Autodesk Inventor part; units mm, degrees
(part 3 of 3)
  circle A2075 centre (2.45, 2.35) radius 0.15
  circle A2076 centre (2.45, 2.05) radius 0.15
  circle A2077 centre (2.45, 1.75) radius 0.15
  circle A2078 centre (2.45, 1.45) radius 0.15
  circle A2079 centre (2.45, 1.15) radius 0.15
  circle A2080 centre (2.45, 0.85) radius 0.15
  circle A2081 centre (2.45, 0.55) radius 0.15
  circle A2082 centre (2.45, 0.25) radius 0.15
  circle A2083 centre (2.45, -0.05) radius 0.15
  circle A2084 centre (2.45, -0.35) radius 0.15
  circle A2085 centre (2.45, -0.65) radius 0.15
  circle A2086 centre (2.45, -0.95) radius 0.15
  circle A2087 centre (2.45, -1.25) radius 0.15
  circle A2088 centre (2.45, -1.55) radius 0.15
  circle A2089 centre (2.45, -1.85) radius 0.15
  circle A2090 centre (2.45, -2.15) radius 0.15
  circle A2091 centre (2.45, -2.45) radius 0.15
  circle A2092 centre (2.45, -2.75) radius 0.15
  circle A2093 centre (2.45, -3.05) radius 0.15
  circle A2094 centre (2.45, -3.35) radius 0.15
  circle A2095 centre (2.45, -3.65) radius 0.15
  circle A2096 centre (2.45, -3.95) radius 0.15
  circle A2097 centre (2.45, -4.25) radius 0.15
  circle A2098 centre (2.45, -4.55) radius 0.15
  circle A2099 centre (2.45, -4.85) radius 0.15
  circle A2100 centre (2.75, 9.85) radius 0.15
  circle A2101 centre (2.75, 9.55) radius 0.15
  circle A2102 centre (2.75, 9.25) radius 0.15
  circle A2103 centre (2.75, 8.95) radius 0.15
  circle A2104 centre (2.75, 8.65) radius 0.15
  circle A2105 centre (2.75, 8.35) radius 0.15
  circle A2106 centre (2.75, 8.05) radius 0.15
  circle A2107 centre (2.75, 7.75) radius 0.15
  circle A2108 centre (2.75, 7.45) radius 0.15
  circle A2109 centre (2.75, 7.15) radius 0.15
  circle A2110 centre (2.75, 6.85) radius 0.15
  circle A2111 centre (2.75, 6.55) radius 0.15
  circle A2112 centre (2.75, 6.25) radius 0.15
  circle A2113 centre (2.75, 5.95) radius 0.15
  circle A2114 centre (2.75, 5.65) radius 0.15
  circle A2115 centre (2.75, 5.35) radius 0.15
  circle A2116 centre (2.75, 5.05) radius 0.15
  circle A2117 centre (2.75, 4.75) radius 0.15
  circle A2118 centre (2.75, 4.45) radius 0.15
  circle A2119 centre (2.75, 4.15) radius 0.15
  circle A2120 centre (2.75, 3.85) radius 0.15
  circle A2121 centre (2.75, 3.55) radius 0.15
  circle A2122 centre (2.75, 3.25) radius 0.15
  circle A2123 centre (2.75, 2.95) radius 0.15
  circle A2124 centre (2.75, 2.65) radius 0.15
  circle A2125 centre (2.75, 2.35) radius 0.15
  circle A2126 centre (2.75, 2.05) radius 0.15
  circle A2127 centre (2.75, 1.75) radius 0.15
  circle A2128 centre (2.75, 1.45) radius 0.15
  circle A2129 centre (2.75, 1.15) radius 0.15
  circle A2130 centre (2.75, 0.85) radius 0.15
  circle A2131 centre (2.75, 0.55) radius 0.15
  circle A2132 centre (2.75, 0.25) radius 0.15
  circle A2133 centre (2.75, -0.05) radius 0.15
  circle A2134 centre (2.75, -0.35) radius 0.15
  circle A2135 centre (2.75, -0.65) radius 0.15
  circle A2136 centre (2.75, -0.95) radius 0.15
  circle A2137 centre (2.75, -1.25) radius 0.15
  circle A2138 centre (2.75, -1.55) radius 0.15
  circle A2139 centre (2.75, -1.85) radius 0.15
  circle A2140 centre (2.75, -2.15) radius 0.15
  circle A2141 centre (2.75, -2.45) radius 0.15
  circle A2142 centre (2.75, -2.75) radius 0.15
  circle A2143 centre (2.75, -3.05) radius 0.15
  circle A2144 centre (2.75, -3.35) radius 0.15
  circle A2145 centre (2.75, -3.65) radius 0.15
  circle A2146 centre (2.75, -3.95) radius 0.15
  circle A2147 centre (2.75, -4.25) radius 0.15
  circle A2148 centre (2.75, -4.55) radius 0.15
  circle A2149 centre (2.75, -4.85) radius 0.15
  circle A2150 centre (3.05, 9.85) radius 0.15
  circle A2151 centre (3.05, 9.55) radius 0.15
  circle A2152 centre (3.05, 9.25) radius 0.15
  circle A2153 centre (3.05, 8.95) radius 0.15
  circle A2154 centre (3.05, 8.65) radius 0.15
  circle A2155 centre (3.05, 8.35) radius 0.15
  circle A2156 centre (3.05, 8.05) radius 0.15
  circle A2157 centre (3.05, 7.75) radius 0.15
  circle A2158 centre (3.05, 7.45) radius 0.15
  circle A2159 centre (3.05, 7.15) radius 0.15
  circle A2160 centre (3.05, 6.85) radius 0.15
  circle A2161 centre (3.05, 6.55) radius 0.15
  circle A2162 centre (3.05, 6.25) radius 0.15
  circle A2163 centre (3.05, 5.95) radius 0.15
  circle A2164 centre (3.05, 5.65) radius 0.15
  circle A2165 centre (3.05, 5.35) radius 0.15
  circle A2166 centre (3.05, 5.05) radius 0.15
  circle A2167 centre (3.05, 4.75) radius 0.15
  circle A2168 centre (3.05, 4.45) radius 0.15
  circle A2169 centre (3.05, 4.15) radius 0.15
  circle A2170 centre (3.05, 3.85) radius 0.15
  circle A2171 centre (3.05, 3.55) radius 0.15
  circle A2172 centre (3.05, 3.25) radius 0.15
  circle A2173 centre (3.05, 2.95) radius 0.15
  circle A2174 centre (3.05, 2.65) radius 0.15
  circle A2175 centre (3.05, 2.35) radius 0.15
  circle A2176 centre (3.05, 2.05) radius 0.15
  circle A2177 centre (3.05, 1.75) radius 0.15
  circle A2178 centre (3.05, 1.45) radius 0.15
  circle A2179 centre (3.05, 1.15) radius 0.15
  circle A2180 centre (3.05, 0.85) radius 0.15
  circle A2181 centre (3.05, 0.55) radius 0.15
  circle A2182 centre (3.05, 0.25) radius 0.15
  circle A2183 centre (3.05, -0.05) radius 0.15
  circle A2184 centre (3.05, -0.35) radius 0.15
  circle A2185 centre (3.05, -0.65) radius 0.15
  circle A2186 centre (3.05, -0.95) radius 0.15
  circle A2187 centre (3.05, -1.25) radius 0.15
  circle A2188 centre (3.05, -1.55) radius 0.15
  circle A2189 centre (3.05, -1.85) radius 0.15
  circle A2190 centre (3.05, -2.15) radius 0.15
  circle A2191 centre (3.05, -2.45) radius 0.15
  circle A2192 centre (3.05, -2.75) radius 0.15
  circle A2193 centre (3.05, -3.05) radius 0.15
  circle A2194 centre (3.05, -3.35) radius 0.15
  circle A2195 centre (3.05, -3.65) radius 0.15
  circle A2196 centre (3.05, -3.95) radius 0.15
  circle A2197 centre (3.05, -4.25) radius 0.15
  circle A2198 centre (3.05, -4.55) radius 0.15
  circle A2199 centre (3.05, -4.85) radius 0.15
  circle A2200 centre (3.35, 9.85) radius 0.15
  circle A2201 centre (3.35, 9.55) radius 0.15
  circle A2202 centre (3.35, 9.25) radius 0.15
  circle A2203 centre (3.35, 8.95) radius 0.15
  circle A2204 centre (3.35, 8.65) radius 0.15
  circle A2205 centre (3.35, 8.35) radius 0.15
  circle A2206 centre (3.35, 8.05) radius 0.15
  circle A2207 centre (3.35, 7.75) radius 0.15
  circle A2208 centre (3.35, 7.45) radius 0.15
  circle A2209 centre (3.35, 7.15) radius 0.15
  circle A2210 centre (3.35, 6.85) radius 0.15
  circle A2211 centre (3.35, 6.55) radius 0.15
  circle A2212 centre (3.35, 6.25) radius 0.15
  circle A2213 centre (3.35, 5.95) radius 0.15
  circle A2214 centre (3.35, 5.65) radius 0.15
  circle A2215 centre (3.35, 5.35) radius 0.15
  circle A2216 centre (3.35, 5.05) radius 0.15
  circle A2217 centre (3.35, 4.75) radius 0.15
  circle A2218 centre (3.35, 4.45) radius 0.15
  circle A2219 centre (3.35, 4.15) radius 0.15
  circle A2220 centre (3.35, 3.85) radius 0.15
  circle A2221 centre (3.35, 3.55) radius 0.15
  circle A2222 centre (3.35, 3.25) radius 0.15
  circle A2223 centre (3.35, 2.95) radius 0.15
  circle A2224 centre (3.35, 2.65) radius 0.15
  circle A2225 centre (3.35, 2.35) radius 0.15
  circle A2226 centre (3.35, 2.05) radius 0.15
  circle A2227 centre (3.35, 1.75) radius 0.15
  circle A2228 centre (3.35, 1.45) radius 0.15
  circle A2229 centre (3.35, 1.15) radius 0.15
  circle A2230 centre (3.35, 0.85) radius 0.15
  circle A2231 centre (3.35, 0.55) radius 0.15
  circle A2232 centre (3.35, 0.25) radius 0.15
  circle A2233 centre (3.35, -0.05) radius 0.15
  circle A2234 centre (3.35, -0.35) radius 0.15
  circle A2235 centre (3.35, -0.65) radius 0.15
  circle A2236 centre (3.35, -0.95) radius 0.15
  circle A2237 centre (3.35, -1.25) radius 0.15
  circle A2238 centre (3.35, -1.55) radius 0.15
  circle A2239 centre (3.35, -1.85) radius 0.15
  circle A2240 centre (3.35, -2.15) radius 0.15
  circle A2241 centre (3.35, -2.45) radius 0.15
  circle A2242 centre (3.35, -2.75) radius 0.15
  circle A2243 centre (3.35, -3.05) radius 0.15
  circle A2244 centre (3.35, -3.35) radius 0.15
  circle A2245 centre (3.35, -3.65) radius 0.15
  circle A2246 centre (3.35, -3.95) radius 0.15
  circle A2247 centre (3.35, -4.25) radius 0.15
  circle A2248 centre (3.35, -4.55) radius 0.15
  circle A2249 centre (3.35, -4.85) radius 0.15
  circle A2250 centre (3.65, 9.85) radius 0.15
  circle A2251 centre (3.65, 9.55) radius 0.15
  circle A2252 centre (3.65, 9.25) radius 0.15
  circle A2253 centre (3.65, 8.95) radius 0.15
  circle A2254 centre (3.65, 8.65) radius 0.15
  circle A2255 centre (3.65, 8.35) radius 0.15
  circle A2256 centre (3.65, 8.05) radius 0.15
  circle A2257 centre (3.65, 7.75) radius 0.15
  circle A2258 centre (3.65, 7.45) radius 0.15
  circle A2259 centre (3.65, 7.15) radius 0.15
  circle A2260 centre (3.65, 6.85) radius 0.15
  circle A2261 centre (3.65, 6.55) radius 0.15
  circle A2262 centre (3.65, 6.25) radius 0.15
  circle A2263 centre (3.65, 5.95) radius 0.15
  circle A2264 centre (3.65, 5.65) radius 0.15
  circle A2265 centre (3.65, 5.35) radius 0.15
  circle A2266 centre (3.65, 5.05) radius 0.15
  circle A2267 centre (3.65, 4.75) radius 0.15
  circle A2268 centre (3.65, 4.45) radius 0.15
  circle A2269 centre (3.65, 4.15) radius 0.15
  circle A2270 centre (3.65, 3.85) radius 0.15
  circle A2271 centre (3.65, 3.55) radius 0.15
  circle A2272 centre (3.65, 3.25) radius 0.15
  circle A2273 centre (3.65, 2.95) radius 0.15
  circle A2274 centre (3.65, 2.65) radius 0.15
  circle A2275 centre (3.65, 2.35) radius 0.15
  circle A2276 centre (3.65, 2.05) radius 0.15
  circle A2277 centre (3.65, 1.75) radius 0.15
  circle A2278 centre (3.65, 1.45) radius 0.15
  circle A2279 centre (3.65, 1.15) radius 0.15
  circle A2280 centre (3.65, 0.85) radius 0.15
  circle A2281 centre (3.65, 0.55) radius 0.15
  circle A2282 centre (3.65, 0.25) radius 0.15
  circle A2283 centre (3.65, -0.05) radius 0.15
  circle A2284 centre (3.65, -0.35) radius 0.15
  circle A2285 centre (3.65, -0.65) radius 0.15
  circle A2286 centre (3.65, -0.95) radius 0.15
  circle A2287 centre (3.65, -1.25) radius 0.15
  circle A2288 centre (3.65, -1.55) radius 0.15
  circle A2289 centre (3.65, -1.85) radius 0.15
  circle A2290 centre (3.65, -2.15) radius 0.15
  circle A2291 centre (3.65, -2.45) radius 0.15
  circle A2292 centre (3.65, -2.75) radius 0.15
  circle A2293 centre (3.65, -3.05) radius 0.15
  circle A2294 centre (3.65, -3.35) radius 0.15
  circle A2295 centre (3.65, -3.65) radius 0.15
  circle A2296 centre (3.65, -3.95) radius 0.15
  circle A2297 centre (3.65, -4.25) radius 0.15
  circle A2298 centre (3.65, -4.55) radius 0.15
  circle A2299 centre (3.65, -4.85) radius 0.15
  circle A2300 centre (3.95, 9.85) radius 0.15
  circle A2301 centre (3.95, 9.55) radius 0.15
  circle A2302 centre (3.95, 9.25) radius 0.15
  circle A2303 centre (3.95, 8.95) radius 0.15
  circle A2304 centre (3.95, 8.65) radius 0.15
  circle A2305 centre (3.95, 8.35) radius 0.15
  circle A2306 centre (3.95, 8.05) radius 0.15
  circle A2307 centre (3.95, 7.75) radius 0.15
  circle A2308 centre (3.95, 7.45) radius 0.15
  circle A2309 centre (3.95, 7.15) radius 0.15
  circle A2310 centre (3.95, 6.85) radius 0.15
  circle A2311 centre (3.95, 6.55) radius 0.15
  circle A2312 centre (3.95, 6.25) radius 0.15
  circle A2313 centre (3.95, 5.95) radius 0.15
  circle A2314 centre (3.95, 5.65) radius 0.15
  circle A2315 centre (3.95, 5.35) radius 0.15
  circle A2316 centre (3.95, 5.05) radius 0.15
  circle A2317 centre (3.95, 4.75) radius 0.15
  circle A2318 centre (3.95, 4.45) radius 0.15
  circle A2319 centre (3.95, 4.15) radius 0.15
  circle A2320 centre (3.95, 3.85) radius 0.15
  circle A2321 centre (3.95, 3.55) radius 0.15
  circle A2322 centre (3.95, 3.25) radius 0.15
  circle A2323 centre (3.95, 2.95) radius 0.15
  circle A2324 centre (3.95, 2.65) radius 0.15
  circle A2325 centre (3.95, 2.35) radius 0.15
  circle A2326 centre (3.95, 2.05) radius 0.15
  circle A2327 centre (3.95, 1.75) radius 0.15
  circle A2328 centre (3.95, 1.45) radius 0.15
  circle A2329 centre (3.95, 1.15) radius 0.15
  circle A2330 centre (3.95, 0.85) radius 0.15
  circle A2331 centre (3.95, 0.55) radius 0.15
  circle A2332 centre (3.95, 0.25) radius 0.15
  circle A2333 centre (3.95, -0.05) radius 0.15
  circle A2334 centre (3.95, -0.35) radius 0.15
  circle A2335 centre (3.95, -0.65) radius 0.15
  circle A2336 centre (3.95, -0.95) radius 0.15
  circle A2337 centre (3.95, -1.25) radius 0.15
  circle A2338 centre (3.95, -1.55) radius 0.15
  circle A2339 centre (3.95, -1.85) radius 0.15
  circle A2340 centre (3.95, -2.15) radius 0.15
  circle A2341 centre (3.95, -2.45) radius 0.15
  circle A2342 centre (3.95, -2.75) radius 0.15
  circle A2343 centre (3.95, -3.05) radius 0.15
  circle A2344 centre (3.95, -3.35) radius 0.15
  circle A2345 centre (3.95, -3.65) radius 0.15
  circle A2346 centre (3.95, -3.95) radius 0.15
  circle A2347 centre (3.95, -4.25) radius 0.15
  circle A2348 centre (3.95, -4.55) radius 0.15
  circle A2349 centre (3.95, -4.85) radius 0.15
  circle A2350 centre (4.25, 9.85) radius 0.15
  circle A2351 centre (4.25, 9.55) radius 0.15
  circle A2352 centre (4.25, 9.25) radius 0.15
  circle A2353 centre (4.25, 8.95) radius 0.15
  circle A2354 centre (4.25, 8.65) radius 0.15
  circle A2355 centre (4.25, 8.35) radius 0.15
  circle A2356 centre (4.25, 8.05) radius 0.15
  circle A2357 centre (4.25, 7.75) radius 0.15
  circle A2358 centre (4.25, 7.45) radius 0.15
  circle A2359 centre (4.25, 7.15) radius 0.15
  circle A2360 centre (4.25, 6.85) radius 0.15
  circle A2361 centre (4.25, 6.55) radius 0.15
  circle A2362 centre (4.25, 6.25) radius 0.15
  circle A2363 centre (4.25, 5.95) radius 0.15
  circle A2364 centre (4.25, 5.65) radius 0.15
  circle A2365 centre (4.25, 5.35) radius 0.15
  circle A2366 centre (4.25, 5.05) radius 0.15
  circle A2367 centre (4.25, 4.75) radius 0.15
  circle A2368 centre (4.25, 4.45) radius 0.15
  circle A2369 centre (4.25, 4.15) radius 0.15
  circle A2370 centre (4.25, 3.85) radius 0.15
  circle A2371 centre (4.25, 3.55) radius 0.15
  circle A2372 centre (4.25, 3.25) radius 0.15
  circle A2373 centre (4.25, 2.95) radius 0.15
  circle A2374 centre (4.25, 2.65) radius 0.15
  circle A2375 centre (4.25, 2.35) radius 0.15
  circle A2376 centre (4.25, 2.05) radius 0.15
  circle A2377 centre (4.25, 1.75) radius 0.15
  circle A2378 centre (4.25, 1.45) radius 0.15
  circle A2379 centre (4.25, 1.15) radius 0.15
  circle A2380 centre (4.25, 0.85) radius 0.15
  circle A2381 centre (4.25, 0.55) radius 0.15
  circle A2382 centre (4.25, 0.25) radius 0.15
  circle A2383 centre (4.25, -0.05) radius 0.15
  circle A2384 centre (4.25, -0.35) radius 0.15
  circle A2385 centre (4.25, -0.65) radius 0.15
  circle A2386 centre (4.25, -0.95) radius 0.15
  circle A2387 centre (4.25, -1.25) radius 0.15
  circle A2388 centre (4.25, -1.55) radius 0.15
  circle A2389 centre (4.25, -1.85) radius 0.15
  circle A2390 centre (4.25, -2.15) radius 0.15
  circle A2391 centre (4.25, -2.45) radius 0.15
  circle A2392 centre (4.25, -2.75) radius 0.15
  circle A2393 centre (4.25, -3.05) radius 0.15
  circle A2394 centre (4.25, -3.35) radius 0.15
  circle A2395 centre (4.25, -3.65) radius 0.15
  circle A2396 centre (4.25, -3.95) radius 0.15
  circle A2397 centre (4.25, -4.25) radius 0.15
  circle A2398 centre (4.25, -4.55) radius 0.15
  circle A2399 centre (4.25, -4.85) radius 0.15
  circle A2400 centre (4.55, 9.85) radius 0.15
  circle A2401 centre (4.55, 9.55) radius 0.15
  circle A2402 centre (4.55, 9.25) radius 0.15
  circle A2403 centre (4.55, 8.95) radius 0.15
  circle A2404 centre (4.55, 8.65) radius 0.15
  circle A2405 centre (4.55, 8.35) radius 0.15
  circle A2406 centre (4.55, 8.05) radius 0.15
  circle A2407 centre (4.55, 7.75) radius 0.15
  circle A2408 centre (4.55, 7.45) radius 0.15
  circle A2409 centre (4.55, 7.15) radius 0.15
  circle A2410 centre (4.55, 6.85) radius 0.15
  circle A2411 centre (4.55, 6.55) radius 0.15
  circle A2412 centre (4.55, 6.25) radius 0.15
  circle A2413 centre (4.55, 5.95) radius 0.15
  circle A2414 centre (4.55, 5.65) radius 0.15
  circle A2415 centre (4.55, 5.35) radius 0.15
  circle A2416 centre (4.55, 5.05) radius 0.15
  circle A2417 centre (4.55, 4.75) radius 0.15
  circle A2418 centre (4.55, 4.45) radius 0.15
  circle A2419 centre (4.55, 4.15) radius 0.15
  circle A2420 centre (4.55, 3.85) radius 0.15
  circle A2421 centre (4.55, 3.55) radius 0.15
  circle A2422 centre (4.55, 3.25) radius 0.15
  circle A2423 centre (4.55, 2.95) radius 0.15
  circle A2424 centre (4.55, 2.65) radius 0.15
  circle A2425 centre (4.55, 2.35) radius 0.15
  circle A2426 centre (4.55, 2.05) radius 0.15
  circle A2427 centre (4.55, 1.75) radius 0.15
  circle A2428 centre (4.55, 1.45) radius 0.15
  circle A2429 centre (4.55, 1.15) radius 0.15
  circle A2430 centre (4.55, 0.85) radius 0.15
  circle A2431 centre (4.55, 0.55) radius 0.15
  circle A2432 centre (4.55, 0.25) radius 0.15
  circle A2433 centre (4.55, -0.05) radius 0.15
  circle A2434 centre (4.55, -0.35) radius 0.15
  circle A2435 centre (4.55, -0.65) radius 0.15
  circle A2436 centre (4.55, -0.95) radius 0.15
  circle A2437 centre (4.55, -1.25) radius 0.15
  circle A2438 centre (4.55, -1.55) radius 0.15
  circle A2439 centre (4.55, -1.85) radius 0.15
  circle A2440 centre (4.55, -2.15) radius 0.15
  circle A2441 centre (4.55, -2.45) radius 0.15
  circle A2442 centre (4.55, -2.75) radius 0.15
  circle A2443 centre (4.55, -3.05) radius 0.15
  circle A2444 centre (4.55, -3.35) radius 0.15
  circle A2445 centre (4.55, -3.65) radius 0.15
  circle A2446 centre (4.55, -3.95) radius 0.15
  circle A2447 centre (4.55, -4.25) radius 0.15
  circle A2448 centre (4.55, -4.55) radius 0.15
  circle A2449 centre (4.55, -4.85) radius 0.15
  circle A2450 centre (4.85, 9.85) radius 0.15
  circle A2451 centre (4.85, 9.55) radius 0.15
  circle A2452 centre (4.85, 9.25) radius 0.15
  circle A2453 centre (4.85, 8.95) radius 0.15
  circle A2454 centre (4.85, 8.65) radius 0.15
  circle A2455 centre (4.85, 8.35) radius 0.15
  circle A2456 centre (4.85, 8.05) radius 0.15
  circle A2457 centre (4.85, 7.75) radius 0.15
  circle A2458 centre (4.85, 7.45) radius 0.15
  circle A2459 centre (4.85, 7.15) radius 0.15
  circle A2460 centre (4.85, 6.85) radius 0.15
  circle A2461 centre (4.85, 6.55) radius 0.15
  circle A2462 centre (4.85, 6.25) radius 0.15
  circle A2463 centre (4.85, 5.95) radius 0.15
  circle A2464 centre (4.85, 5.65) radius 0.15
  circle A2465 centre (4.85, 5.35) radius 0.15
  circle A2466 centre (4.85, 5.05) radius 0.15
  circle A2467 centre (4.85, 4.75) radius 0.15
  circle A2468 centre (4.85, 4.45) radius 0.15
  circle A2469 centre (4.85, 4.15) radius 0.15
  circle A2470 centre (4.85, 3.85) radius 0.15
  circle A2471 centre (4.85, 3.55) radius 0.15
  circle A2472 centre (4.85, 3.25) radius 0.15
  circle A2473 centre (4.85, 2.95) radius 0.15
  circle A2474 centre (4.85, 2.65) radius 0.15
  circle A2475 centre (4.85, 2.35) radius 0.15
  circle A2476 centre (4.85, 2.05) radius 0.15
  circle A2477 centre (4.85, 1.75) radius 0.15
  circle A2478 centre (4.85, 1.45) radius 0.15
  circle A2479 centre (4.85, 1.15) radius 0.15
  circle A2480 centre (4.85, 0.85) radius 0.15
  circle A2481 centre (4.85, 0.55) radius 0.15
  circle A2482 centre (4.85, 0.25) radius 0.15
  circle A2483 centre (4.85, -0.05) radius 0.15
  circle A2484 centre (4.85, -0.35) radius 0.15
  circle A2485 centre (4.85, -0.65) radius 0.15
  circle A2486 centre (4.85, -0.95) radius 0.15
  circle A2487 centre (4.85, -1.25) radius 0.15
  circle A2488 centre (4.85, -1.55) radius 0.15
  circle A2489 centre (4.85, -1.85) radius 0.15
  circle A2490 centre (4.85, -2.15) radius 0.15
  circle A2491 centre (4.85, -2.45) radius 0.15
  circle A2492 centre (4.85, -2.75) radius 0.15
  circle A2493 centre (4.85, -3.05) radius 0.15
  circle A2494 centre (4.85, -3.35) radius 0.15
  circle A2495 centre (4.85, -3.65) radius 0.15
  circle A2496 centre (4.85, -3.95) radius 0.15
  circle A2497 centre (4.85, -4.25) radius 0.15
  circle A2498 centre (4.85, -4.55) radius 0.15
  circle A2499 centre (4.85, -4.85) radius 0.15
  line L14 (-9.55, 10) -> (-9.55, -10)
  line L15 (-9.25, 10) -> (-9.25, -10)
  line L16 (-8.95, 10) -> (-8.95, -10)
  line L17 (-8.65, 10) -> (-8.65, -10)
  line L18 (-8.35, 10) -> (-8.35, -10)
  line L19 (-8.05, 10) -> (-8.05, -10)
  line L20 (-7.75, 10) -> (-7.75, -10)
  line L21 (-7.45, 10) -> (-7.45, -10)
  line L22 (-7.15, 10) -> (-7.15, -10)
  line L23 (-6.85, 10) -> (-6.85, -10)
  line L24 (-6.55, 10) -> (-6.55, -10)
  line L25 (-6.25, 10) -> (-6.25, -10)
  line L26 (-5.95, 10) -> (-5.95, -10)
  line L27 (-5.65, 10) -> (-5.65, -10)
  line L28 (-5.35, 10) -> (-5.35, -10)
  line L29 (-5.05, 10) -> (-5.05, -10)
  line L30 (-4.75, 10) -> (-4.75, -10)
  line L31 (-4.45, 10) -> (-4.45, -10)
  line L32 (-4.15, 10) -> (-4.15, -10)
  line L33 (-3.85, 10) -> (-3.85, -10)
  line L34 (-3.55, 10) -> (-3.55, -10)
  line L35 (-3.25, 10) -> (-3.25, -10)
  line L36 (-2.95, 10) -> (-2.95, -10)
  line L37 (-2.65, 10) -> (-2.65, -10)
  line L38 (-2.35, 10) -> (-2.35, -10)
  line L39 (-2.05, 10) -> (-2.05, -10)
  line L40 (-1.75, 10) -> (-1.75, -10)
  line L41 (-1.45, 10) -> (-1.45, -10)
  line L42 (-1.15, 10) -> (-1.15, -10)
  line L43 (-0.85, 10) -> (-0.85, -10)
  line L44 (-0.55, 10) -> (-0.55, -10)
  line L45 (-0.25, 10) -> (-0.25, -10)
  line L46 (0.05, 10) -> (0.05, -10)
  line L47 (0.35, 10) -> (0.35, -10)
  line L48 (0.65, 10) -> (0.65, -10)
  line L49 (0.95, 10) -> (0.95, -10)
  line L50 (1.25, 10) -> (1.25, -10)
  line L51 (1.55, 10) -> (1.55, -10)
  line L52 (1.85, 10) -> (1.85, -10)
  line L53 (2.15, 10) -> (2.15, -10)
  line L54 (2.45, 10) -> (2.45, -10)
  line L55 (2.75, 10) -> (2.75, -10)
  line L56 (3.05, 10) -> (3.05, -10)
  line L57 (3.35, 10) -> (3.35, -10)
  line L58 (3.65, 10) -> (3.65, -10)
  line L59 (3.95, 10) -> (3.95, -10)
  line L60 (4.25, 10) -> (4.25, -10)
  line L61 (4.55, 10) -> (4.55, -10)
  line L62 (4.85, 10) -> (4.85, -10)
  point P0 (0, 0)
  point P1 (-9.85, 9.7)
  point P2 (-9.85, 8.5)
  point P3 (-9.85, 8.8)
  point P4 (-9.85, 8.8)
  point P5 (-9.85, 8.8)
  point P6 (-9.85, 9.1)
  point P7 (-9.85, 9.1)
  point P8 (-9.85, 9.1)
  point P9 (-9.85, 9.4)
  point P10 (-9.85, 9.4)
  point P11 (-9.85, 9.4)
  point P12 (-9.85, 9.7)
  dimension "d0" = 20
  dimension "d1" = 0.15
  dimension "d2" = 20
  dimension "d3" = 0.15
  dimension "d4" = 20
  dimension "d5" = 0.3
  dimension "d13" = 0.3
  dimension "d16" = 0.3
  dimension "d21" = 0.3
  constraints: 2500 centre point, 126 end point, 55 point on line, 5 horizontal, 4 parallel, 3 perpendicular, 2 vertical, 5196 other
  measures "d0" distance of L0.start L0.end
  measures "d1" distance of L0.start L6.end
  measures "d2" distance of L6.end L7.end
  measures "d3" distance of L0.start L8.end
  measures "d4" distance of L8.end L9.end
  measures "d5" diameter of A0
  measures "d13" distance of A0.centre A1.centre
  measures "d16" distance of A0.centre A50.centre
  measures "d21" distance of L8.end L14.start
revolve "Umdrehung1" add sketch "Skizze1" angle 180 about axis through (-9.85, 10, 0) along (0, 1, 0) picked at (-9.9476, 9.8655) picked at (-9.8948, 9.762) picked at (-9.8206, 9.5905) picked at (-9.8794, 9.2095) picked at (-9.8976, 8.9655) picked at (-9.913, 8.637) contours L9 L7 A0 | L7 L9 A0 | A1 L9 | A2 L9 | A3 L9 | A4 L9
sketch "Skizze2" plane through (-9.85, 9.85, 0) normal (0, 0, 1) x (1, 0, 0)
  circle A0 centre (0, 0) radius 0.15 projected
  line L0 (0, 0) -> (-0.15, 0)
  line L1 (-0.15, 0) -> (-0.15, 0.15)
  line L2 (-0.15, 0.15) -> (0, 0.15)
  line L3 (0, 0.15) -> (0, 0)
  line L4 (-0.15, 0.15) -> (14.85, 0.15)
  line L5 (14.85, 0.15) -> (14.85, -14.85)
  line L6 (14.85, -14.85) -> (-0.15, -14.85)
  line L7 (-0.15, -14.85) -> (-0.15, 0.15)
  point P0 (9.85, -9.85)
  point P1 (0, 0.15)
  point P2 (-0.15, 0)
  point P3 (-0.15, 0)
  point P4 (0, 0.15)
  dimension "d7" = 15
  dimension "d8" = 15
  constraints: 16 end point, 4 parallel, 2 horizontal, 2 perpendicular, 1 other
  measures "d7" distance of L5.end L6.end
  measures "d8" distance of L4.end L5.end
extrude "Extrusion1" [suppressed]
